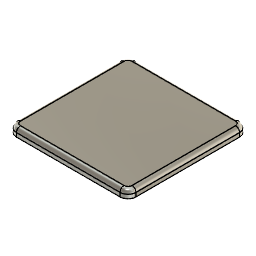
p4-plant_stand (Autodesk Fusion 360 design; units mm, degrees)
part number: 2025-10-23-22-53-58-743
Autodesk Fusion 360 part; units mm, degrees
sketch "Sketch2" plane through (0, -66.1791, -11.6692) normal (0, -0.984808, -0.173648) x (1, 0, 0)
  line L0 (-65, 123.5461) -> (-65, 22.0034)
  line L1 (-65, 22.0034) -> (65, 22.0034)
  line L2 (65, 22.0034) -> (65, 123.5461)
  line L3 (65, 123.5461) -> (55, 123.5461)
  line L4 (55, 123.5461) -> (-65, 123.5461)
  circle A0 centre (25, 62.0034) radius 0
  dimension "d1" = 0
  dimension "d2" = 40
  dimension "d3" = 40
  measures "d1" diameter of A0
  measures "d2" distance of L2 A0.centre
  measures "d3" distance of L1 A0.centre
sketch "Sketch1" plane through (0, 0, 0) normal (0, 0, 1) x (1, 0, 0)
  line L0 (75, 75) -> (-75, 75)
  line L1 (-75, 75) -> (-75, -75)
  line L2 (-75, -75) -> (75, -75)
  line L3 (75, -75) -> (75, 75)
  line L4 (75, 75) -> (-75, -75) construction
  line L5 (-75, 75) -> (75, -75) construction
  dimension "d17" = 150
  dimension "d18" = 150
  constraint horizontal L0
  constraint perpendicular L0 L1
  constraint parallel L0 L2
  constraint parallel L1 L3
  constraint coincident L4 origin
  constraint coincident L5 origin
  measures "d17" distance of L1.end L2.end
  measures "d18" distance of L0.end L1.end
extrude "Extrude1" add sketch "Sketch1" along normal blind 10
fillet "Fillet1" radius 10 4 edges at (-75, -75, 5) (75, -75, 5) (75, 75, 5) (-75, 75, 5)
fillet "Fillet1" radius 5 4 edges at (75, 0, 10) (0, 75, 10) (-75, 0, 10) (0, -75, 10)
extrude "Extrude2" [suppressed]
equation "d17 = standwidth"
equation "d18 = standwidth"
equation "d19 = standheight"
equation "standwidth = 150 mm"
equation "standheight = 10 mm"
equation "d1 = speakerhole_f"
